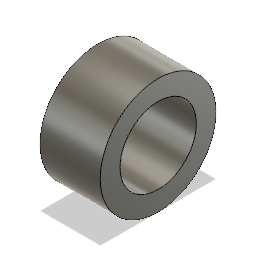
_jj.35ade954-a849-465f-ba52-b935902dbde0 (Autodesk Fusion 360 design; units mm, degrees)
Autodesk Fusion 360 part; units mm, degrees
sketch "Sketch1" plane through (0, 0, 0) normal (1, 0, 0) x (0, 0, -1)
  circle A0 centre (-25.8288, 17.5342) radius 14.3842
  circle A1 centre (-25.8288, 17.5342) radius 9.4717
extrude "Extrude1" add sketch "Sketch1" along normal blind 15
